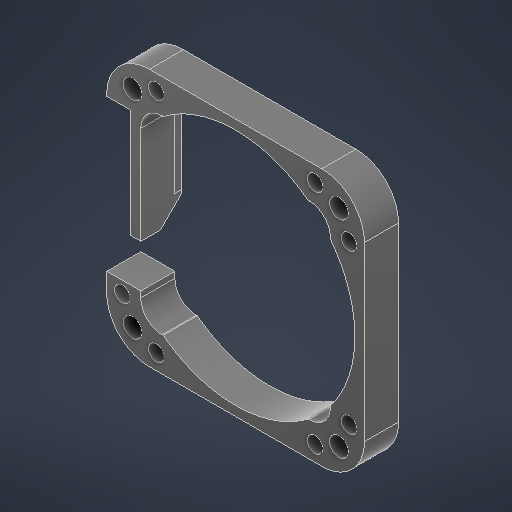
# Autodesk Inventor part: encoder_spacer
Saved by Autodesk Inventor 2026.1 (Build 301233000, 233)
## iProperties
Created: 2026-05-19
Part Number: encoder_spacer
Material: ABS Plastic
Document SubType Name: Modeling
Designer: aaron
Density: 1.06 g/cm^3
Appearance: Smooth - White
Author: aaron
Autodesk Inventor part; units mm, degrees
ref_plane "YZ Plane" through (0, 0, 0) normal (1, 0, 0) x (0, 1, 0)
ref_plane "XZ Plane" through (0, 0, 0) normal (0, 1, 0) x (-1, 0, 0)
ref_plane "XY Plane" through (0, 0, 0) normal (0, 0, 1) x (1, 0, 0)
sketch "Sketch1" plane through (0, 0, 0) normal (0, 0, 1) x (1, 0, 0)
  line L0 (20, 0) -> (101, 0)
  line L1 (121, 20) -> (121, 101)
  line L2 (101, 121) -> (20, 121)
  line L3 (0, 101) -> (0, 20)
  arc A0 (20, 121) -> (0, 101) centre (20, 101) ccw
  arc A1 (121, 101) -> (101, 121) centre (101, 101) ccw
  arc A2 (101, 0) -> (121, 20) centre (101, 20) ccw
  arc A3 (0, 20) -> (20, 0) centre (20, 20) ccw
  point P0 (0, 0)
  point P1 (121, 0)
  point P2 (0, 121)
  dimension "d0" = 121
  dimension "d1" = 121
  dimension "d2" = 20
  constraints: 8 end point, 8 point on circle, 8 tangent, 6 point on line, 4 centre point, 3 equal radius, 2 parallel, 1 horizontal, 1 perpendicular
  measures "d0" distance of point (0, 121) point (0, 0)
  measures "d1" distance of point (0, 0) point (121, 0)
  measures "d2" radius of A0
extrude "Extrusion1" add sketch "Sketch1" against normal blind 12
sketch "Sketch2" plane through (0, 0, -12) normal (0, 0, -1) x (-1, 0, 0)
  circle A0 centre (-11.9934, 108.9934) radius 2.65 projected
  circle A1 centre (-7.2551, 97.7825) radius 2.15 projected
  circle A2 centre (-23.2175, 113.7449) radius 2.15 projected
  circle A3 centre (-7.2551, 23.2175) radius 2.15 projected
  circle A4 centre (-12, 12) radius 2.65 projected
  circle A5 centre (-12, 12) radius 2.65 projected
  circle A6 centre (-23.2175, 7.2551) radius 2.15 projected
  circle A7 centre (-97.7825, 7.2551) radius 2.15 projected
  circle A8 centre (-109, 12) radius 2.65 projected
  circle A9 centre (-113.7449, 23.2175) radius 2.15 projected
  circle A10 centre (-113.7449, 97.7825) radius 2.15 projected
  circle A11 centre (-109, 109) radius 2.65 projected
  circle A12 centre (-97.7825, 113.7449) radius 2.15 projected
  point P0 (0, 0)
extrude "Extrusion2" cut sketch "Sketch2" against normal through all
sketch "Sketch3" plane through (0, 0, 0) normal (0, 0, 1) x (1, 0, 0)
  circle A0 centre (113.7449, 97.7825) radius 2.15 projected
  circle A1 centre (7.2551, 23.2175) radius 2.15 projected
  circle A2 centre (109, 12) radius 2.65 projected
  circle A3 centre (97.7825, 7.2551) radius 2.15 projected
  circle A4 centre (7.2551, 97.7825) radius 2.15 projected
  circle A5 centre (109, 109) radius 2.65 projected
  circle A6 centre (23.2175, 113.7449) radius 2.15 projected
  circle A7 centre (12, 12) radius 2.65 projected
  circle A8 centre (113.7449, 23.2175) radius 2.15 projected
  circle A9 centre (23.2175, 7.2551) radius 2.15 projected
  circle A10 centre (11.9934, 108.9934) radius 2.65 projected
  circle A11 centre (97.7825, 113.7449) radius 2.15 projected
  arc A12 (101, 0) -> (121, 20) centre (101, 20) ccw projected
  line L0 (121, 20) -> (121, 101) projected
  arc A13 (121, 101) -> (101, 121) centre (101, 101) ccw projected
  line L1 (101, 121) -> (20, 121) projected
  arc A14 (20, 121) -> (0, 101) centre (20, 101) ccw projected
  line L2 (0, 101) -> (0, 20) projected
  arc A15 (0, 20) -> (20, 0) centre (20, 20) ccw projected
  line L3 (20, 0) -> (101, 0) projected
  line L4 (16, 105) -> (105, 105)
  line L5 (105, 105) -> (105, 16)
  line L6 (105, 16) -> (16, 16)
  line L7 (16, 16) -> (16, 105)
  point P0 (0, 0)
  dimension "d7" = 16
  constraints: 8 end point, 3 other
  measures "d7" distance between parallel lines of L1 L4
extrude "Extrusion3" cut sketch "Sketch3" against normal through all contours L4 L5 L6 L7
fillet "Fillet1" radius 10 4 edges at (16, 105, -6) (105, 105, -6) (105, 16, -6) (16, 16, -6)
sketch "Sketch4" plane through (0, 0, -12) normal (0, 0, -1) x (-1, 0, 0)
  circle A0 centre (-95.0481, 68.0117) radius 1.25 projected
  circle A1 centre (-25.9519, 52.9883) radius 1.25 projected
  circle A2 centre (-68.0117, 25.9519) radius 1.25 projected
  circle A3 centre (-52.9883, 95.0481) radius 1.25 projected
  circle A4 centre (-81.3827, 73.8228) radius 0.8 projected
  circle A5 centre (-29.8334, 29.1758) radius 1.25 projected
  circle A6 centre (-33.3827, 73.8163) radius 0.8 projected
  circle A7 centre (-81.3783, 105.8228) radius 0.8 projected
  circle A8 centre (-93.8334, 29.1845) radius 1.25 projected
  circle A9 centre (-33.3783, 105.8163) radius 0.8 projected
  circle A10 centre (-97.7752, 113.75) radius 2.15 projected
  circle A11 centre (-108.9934, 109.0066) radius 2.65 projected
  circle A12 centre (-11.9934, 108.9934) radius 2.65 projected
  circle A13 centre (-113.75, 23.2248) radius 2.15 projected
  circle A14 centre (-109.0066, 12.0066) radius 2.65 projected
  circle A15 centre (-23.2248, 7.25) radius 2.15 projected
  circle A16 centre (-12.0066, 11.9934) radius 2.65 projected
  circle A17 centre (-113.7398, 97.7897) radius 2.15 projected
  circle A18 centre (-23.2103, 113.7398) radius 2.15 projected
  circle A19 centre (-97.7897, 7.2602) radius 2.15 projected
  circle A20 centre (-7.2602, 23.2103) radius 2.15 projected
  line L0 (-1.0042, 29.9919) -> (-0.0043, 28.9917) projected
  line L1 (-1.0042, 29.9919) -> (-16.0042, 29.9939) projected
  line L2 (-16.0042, 29.9939) -> (-15.9945, 100.9939) projected
  line L3 (-15.9945, 100.9939) -> (-0.9945, 100.9919) projected
  line L4 (-0.0193, 101.9914) -> (-0.9945, 100.9919) projected
  arc A21 (-0.0193, 101.9914) -> (-19.9917, 120.9945) centre (-19.9945, 100.9945) ccw projected
  line L5 (-26.1793, 120.9953) -> (-19.9917, 120.9945) projected
  arc A22 (-26.1793, 120.9953) -> (-32.1801, 114.9961) centre (-26.1801, 114.9953) ccw projected
  line L6 (-32.1801, 114.9961) -> (-32.1804, 113.0461) projected
  line L7 (-32.1804, 113.0461) -> (-35.3604, 113.0466) projected
  line L8 (-35.3604, 113.0466) -> (-35.3601, 114.6366) projected
  line L9 (-35.3601, 114.6366) -> (-85.6251, 114.6434) projected
  line L10 (-85.6251, 114.6434) -> (-85.6253, 113.0534) projected
  line L11 (-85.6253, 113.0534) -> (-88.8053, 113.0539) projected
  line L12 (-88.8053, 113.0539) -> (-88.805, 115.0039) projected
  arc A23 (-88.805, 115.0039) -> (-94.8042, 121.0047) centre (-94.805, 115.0047) ccw projected
  line L13 (-100.9917, 121.0055) -> (-94.8042, 121.0047) projected
  arc A24 (-100.9917, 121.0055) -> (-120.9945, 101.0083) centre (-100.9945, 101.0055) ccw projected
  line L14 (-120.9953, 94.8207) -> (-120.9945, 101.0083) projected
  arc A25 (-120.9953, 94.8207) -> (-114.9961, 88.8199) centre (-114.9953, 94.8199) ccw projected
  line L15 (-114.9961, 88.8199) -> (-113.0461, 88.8196) projected
  line L16 (-113.0461, 88.8196) -> (-113.0466, 85.6396) projected
  line L17 (-113.0466, 85.6396) -> (-114.6366, 85.6399) projected
  line L18 (-114.6366, 85.6399) -> (-114.6434, 35.3749) projected
  line L19 (-114.6434, 35.3749) -> (-113.0534, 35.3747) projected
  line L20 (-113.0534, 35.3747) -> (-113.0539, 32.1947) projected
  line L21 (-113.0539, 32.1947) -> (-115.0039, 32.195) projected
  arc A26 (-115.0039, 32.195) -> (-121.0047, 26.1958) centre (-115.0047, 26.195) ccw projected
  line L22 (-121.0055, 20.0083) -> (-121.0047, 26.1958) projected
  arc A27 (-121.0055, 20.0083) -> (-101.0083, 0.0055) centre (-101.0055, 20.0055) ccw projected
  line L23 (-94.8207, 0.0047) -> (-101.0083, 0.0055) projected
  arc A28 (-94.8207, 0.0047) -> (-88.8199, 6.0039) centre (-94.8199, 6.0047) ccw projected
  line L24 (-88.8199, 6.0039) -> (-88.8196, 7.9539) projected
  line L25 (-88.8196, 7.9539) -> (-85.6396, 7.9534) projected
  line L26 (-85.6396, 7.9534) -> (-85.6399, 6.3634) projected
  line L27 (-85.6399, 6.3634) -> (-35.3749, 6.3566) projected
  line L28 (-35.3749, 6.3566) -> (-35.3747, 7.9466) projected
  line L29 (-35.3747, 7.9466) -> (-32.1947, 7.9461) projected
  line L30 (-32.1947, 7.9461) -> (-32.195, 5.9961) projected
  arc A29 (-32.195, 5.9961) -> (-26.1958, -0.0047) centre (-26.195, 5.9953) ccw projected
  line L31 (-20.0083, -0.0055) -> (-26.1958, -0.0047) projected
  arc A30 (-20.0083, -0.0055) -> (-0.0055, 19.9917) centre (-20.0055, 19.9945) ccw projected
  line L32 (-0.0043, 28.9917) -> (-0.0055, 19.9917) projected
  line L33 (-105, 26) -> (-105, 95) projected
  arc A31 (-95, 105) -> (-105, 95) centre (-95, 95) ccw projected
  line L34 (-95, 105) -> (-26, 105) projected
  arc A32 (-16, 95) -> (-26, 105) centre (-26, 95) ccw projected
  line L35 (-16, 95) -> (-16, 26) projected
  arc A33 (-26, 16) -> (-16, 26) centre (-26, 26) ccw projected
  line L36 (-26, 16) -> (-95, 16) projected
  arc A34 (-105, 26) -> (-95, 16) centre (-95, 26) ccw projected
  circle A35 centre (-113.7449, 97.7825) radius 2.15 projected
  circle A36 centre (-7.2551, 23.2175) radius 2.15 projected
  circle A37 centre (-109, 12) radius 2.65 projected
  circle A38 centre (-97.7825, 7.2551) radius 2.15 projected
  circle A39 centre (-7.2551, 97.7825) radius 2.15 projected
  circle A40 centre (-109, 109) radius 2.65 projected
  circle A41 centre (-23.2175, 113.7449) radius 2.15 projected
  circle A42 centre (-12, 12) radius 2.65 projected
  circle A43 centre (-113.7449, 23.2175) radius 2.15 projected
  circle A44 centre (-23.2175, 7.2551) radius 2.15 projected
  circle A45 centre (-11.9934, 108.9934) radius 2.65 projected
  circle A46 centre (-97.7825, 113.7449) radius 2.15 projected
  arc A47 (-121, 20) -> (-101, 0) centre (-101, 20) ccw projected
  line L37 (-101, 0) -> (-20, 0) projected
  arc A48 (-20, 0) -> (0, 20) centre (-20, 20) ccw projected
  line L38 (0, 20) -> (0, 101) projected
  arc A49 (0, 101) -> (-20, 121) centre (-20, 101) ccw projected
  line L39 (-20, 121) -> (-101, 121) projected
  arc A50 (-101, 121) -> (-121, 101) centre (-101, 101) ccw projected
  line L40 (-121, 101) -> (-121, 20) projected
  line L41 (-0.0043, 28.9917) -> (0.0136, 28.9917)
  point P0 (0, 0)
  point P1 (0, 28.9917)
  point P2 (-0.0243, 101.9863)
  point P3 (-16, 60.497)
  point P4 (-16, 29.9939)
  constraints: 2 end point, 1 horizontal
extrude "Extrusion4" add sketch "Sketch4" along normal blind 3.18 contours L1 L35 L2 L3 L4 A49 L38 L41 L0
sketch "Sketch5" plane through (0, 20, 0) normal (-1, 0, 0) x (0, 0, 1)
  line L0 (-15.18, 80.9939) -> (-15.18, 40.497) projected
  line L1 (10.47, 25) -> (-15.18, 25)
  line L2 (-15.18, 25) -> (-15.18, 80)
  line L3 (-15.18, 80) -> (10.47, 80)
  line L4 (10.47, 80) -> (10.47, 25)
  line L5 (0, 81) -> (0, 0) projected
  line L6 (0, 81) -> (-15.18, 81) projected
  point P0 (0, -20)
  dimension "d13" = 25.65
  dimension "d14" = 55
  dimension "d17" = 10.47
  dimension "d18" = 1
  constraints: 8 end point, 2 parallel, 1 horizontal, 1 perpendicular, 1 point on line
  measures "d13" distance between parallel lines of L4 L2
  measures "d14" distance of L3.end L1.start
  measures "d17" distance between parallel lines of L5 L4
  measures "d18" distance between parallel lines of L6 L3
extrude "Extrusion5" cut sketch "Sketch5" against normal blind 11.35
sketch "Sketch6" plane through (0, 20, -12) normal (-1, 0, 0) x (0, 0, 1)
  line L0 (12, 80) -> (12, 25) projected
  line L1 (12, 25) -> (-7.547, 25)
  line L2 (-7.547, 25) -> (-7.547, 8.8174)
  line L3 (-7.547, 8.8174) -> (12, 8.8174)
  line L4 (12, 8.8174) -> (12, 25)
  point P0 (12, -20)
  constraints: 8 end point, 2 parallel, 1 horizontal, 1 perpendicular
extrude "Extrusion6" cut sketch "Sketch6" against normal blind 30
sketch "Sketch7" plane through (0, 0, 0) normal (0, 0, 1) x (1, 0, 0)
  circle A0 centre (60.5, 60.5) radius 56
  line L0 (26, 105) -> (95, 105) projected
  line L1 (95, 16) -> (26, 16) projected
  line L2 (105, 95) -> (105, 26) projected
  line L3 (16, 45) -> (16, 95) projected
  point P0 (0, 0)
  point P1 (26.5037, 105)
  point P2 (94.4963, 105)
  point P3 (105, 94.4963)
  point P4 (105, 26.5037)
  point P5 (94.4963, 16)
  point P6 (26.5037, 16)
  dimension "d23" = 89
  dimension "d24" = 89
  dimension "d25" = 44.5
  dimension "d26" = 44.5
  dimension "d27" = 112
  constraints: 1 centre point
  measures "d23" distance between parallel lines of L0 L1
  measures "d24" distance between parallel lines of L2 L3
  measures "d25" distance from line of L1 A0.centre
  measures "d26" distance from line of L2 A0.centre
  measures "d27" diameter of A0
extrude "Extrusion7" cut sketch "Sketch7" against normal through all contours A0 L2 | L0 A0 | A0 L1
sketch "Sketch8" plane through (0, 0, 0) normal (0, 0, 1) x (1, 0, 0)
  circle A0 centre (23.2175, 7.2551) radius 2.15 projected
  circle A1 centre (23.2175, 7.2551) radius 3.6
  circle A2 centre (7.2551, 23.2175) radius 2.15 projected
  circle A3 centre (7.2551, 23.2175) radius 3.6
  circle A4 centre (23.2175, 113.7449) radius 2.15 projected
  circle A5 centre (23.2175, 113.7449) radius 3.6
  circle A6 centre (97.7825, 113.7449) radius 2.15 projected
  circle A7 centre (97.7825, 113.7449) radius 3.6
  circle A8 centre (113.7449, 97.7825) radius 2.15 projected
  circle A9 centre (113.7449, 97.7825) radius 3.6
  circle A10 centre (113.7449, 23.2175) radius 2.15 projected
  circle A11 centre (113.7449, 23.2175) radius 3.6
  circle A12 centre (97.7825, 7.2551) radius 2.15 projected
  circle A13 centre (97.7825, 7.2551) radius 3.6
  point P0 (0, 0)
  dimension "d30" = 7.2
  dimension "d31" = 7.2
  dimension "d32" = 7.2
  dimension "d33" = 7.2
  dimension "d34" = 7.2
  dimension "d35" = 7.2
  dimension "d36" = 7.2
  constraints: 7 centre point, 7 coincident
  measures "d30" diameter of A13
  measures "d31" diameter of A1
  measures "d32" diameter of A11
  measures "d33" diameter of A9
  measures "d34" diameter of A7
  measures "d35" diameter of A5
  measures "d36" diameter of A3
extrude "Extrusion8" cut sketch "Sketch8" against normal blind 4 contours A0 | A1 | A2 | A3 | A4 | A5 | A6 | A7 | A8 | A9 | A10 | A11 | A12 | A13
chamfer "Chamfer1" distance 1.45 angle 45 7 edges at (25.3675, 7.2551, -4) (9.4051, 23.2175, -4) (99.9325, 7.2551, -4) (115.8949, 23.2175, -4) (115.8949, 97.7825, -4) (99.9325, 113.7449, -4) (25.3675, 113.7449, -4)
sketch "Sketch9" plane through (0, 0, 0) normal (0, 0, 1) x (1, 0, 0)
  circle A0 centre (11.9934, 108.9934) radius 2.65 projected
  circle A1 centre (12, 12) radius 2.65 projected
  circle A2 centre (109, 12) radius 2.65 projected
  circle A3 centre (109, 109) radius 2.65 projected
  circle A4 centre (11.9934, 108.9934) radius 4.35
  circle A5 centre (109, 109) radius 4.35
  circle A6 centre (109, 12) radius 4.35
  circle A7 centre (12, 12) radius 4.35
  point P0 (0, 0)
  dimension "d42" = 8.7
  dimension "d43" = 8.7
  dimension "d44" = 8.7
  dimension "d45" = 8.7
  constraints: 4 centre point, 4 coincident
  measures "d42" diameter of A4
  measures "d43" diameter of A7
  measures "d44" diameter of A6
  measures "d45" diameter of A5
extrude "Extrusion9" cut sketch "Sketch9" against normal blind 5.2
chamfer "Chamfer2" distance 1.7 angle 45 4 edges at (14.65, 12, -5.2) (111.65, 12, -5.2) (111.65, 109, -5.2) (14.6434, 108.9934, -5.2)
sketch "Sketch10" plane through (0, 0, 0) normal (0, 0, 1) x (1, 0, 0)
  circle A0 centre (12, 12) radius 4.35 projected
  circle A1 centre (109, 109) radius 4.35 projected
  circle A2 centre (109, 12) radius 4.35 projected
  circle A3 centre (11.9934, 108.9934) radius 4.35 projected
  circle A4 centre (97.7825, 7.2551) radius 3.6 projected
  circle A5 centre (23.2175, 113.7449) radius 3.6 projected
  circle A6 centre (113.7449, 23.2175) radius 3.6 projected
  circle A7 centre (23.2175, 7.2551) radius 3.6 projected
  circle A8 centre (97.7825, 113.7449) radius 3.6 projected
  circle A9 centre (113.7449, 97.7825) radius 3.6 projected
  circle A10 centre (7.2551, 23.2175) radius 3.6 projected
  arc A11 (94.4963, 105) -> (26.5037, 105) centre (60.5, 60.5) ccw projected
  line L0 (94.4963, 105) -> (95, 105) projected
  arc A12 (105, 95) -> (95, 105) centre (95, 95) ccw projected
  line L1 (105, 95) -> (105, 94.4963) projected
  arc A13 (105, 26.5037) -> (105, 94.4963) centre (60.5, 60.5) ccw projected
  line L2 (105, 26.5037) -> (105, 26) projected
  arc A14 (95, 16) -> (105, 26) centre (95, 26) ccw projected
  line L3 (95, 16) -> (94.4963, 16) projected
  arc A15 (26.5037, 16) -> (94.4963, 16) centre (60.5, 60.5) ccw projected
  line L4 (26.5037, 16) -> (26, 16) projected
  arc A16 (16, 26) -> (26, 16) centre (26, 26) ccw projected
  line L5 (16, 26) -> (16, 28.8174) projected
  line L6 (16, 28.8174) -> (0, 28.8174) projected
  line L7 (0, 28.8174) -> (0, 20) projected
  arc A17 (0, 20) -> (20, 0) centre (20, 20) ccw projected
  line L8 (20, 0) -> (101, 0) projected
  arc A18 (101, 0) -> (121, 20) centre (101, 20) ccw projected
  line L9 (121, 20) -> (121, 101) projected
  arc A19 (121, 101) -> (101, 121) centre (101, 101) ccw projected
  line L10 (101, 121) -> (20, 121) projected
  arc A20 (20, 121) -> (0, 101) centre (20, 101) ccw projected
  line L11 (0, 101) -> (0, 100) projected
  line L12 (0, 100) -> (11.35, 100) projected
  line L13 (11.35, 100) -> (11.35, 45) projected
  line L14 (11.35, 45) -> (16, 45) projected
  line L15 (16, 45) -> (16, 95) projected
  arc A21 (26, 105) -> (16, 95) centre (26, 95) ccw projected
  line L16 (26, 105) -> (26.5037, 105) projected
  point P0 (0, 0)
extrude "Extrusion10" add sketch "Sketch10" along normal blind 4
chamfer "Chamfer3" distance 14 angle 45 1 edges at (13.675, 45, -15.18)
sketch "Sketch11" plane through (11.35, 45, 4) normal (0, -1, 0) x (1, 0, 0)
  line L0 (17.408, -26.9807) -> (-20.349, -26.9807)
  line L1 (-20.349, -26.9807) -> (-20.349, 7.2541)
  line L2 (-20.349, 7.2541) -> (17.408, 7.2541)
  line L3 (17.408, 7.2541) -> (17.408, -26.9807)
  point P0 (-11.35, -4)
  constraints: 8 end point, 2 parallel, 1 horizontal, 1 perpendicular
extrude "Extrusion11" cut sketch "Sketch11" against normal blind 4
equation "\"d25\" = 0.5 * d23"
equation "\"d26\" = 0.5 * d24"
equation "\"d31\" = d30"
equation "\"d32\" = d30"
equation "\"d33\" = d30"
equation "\"d34\" = d30"
equation "\"d35\" = d30"
equation "\"d36\" = d30"
equation "\"d43\" = d42"
equation "\"d44\" = d42"
equation "\"d45\" = d42"
body "Solid1"
